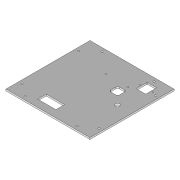
# Autodesk Inventor part: BREEZE-M09
Saved by Autodesk Inventor 2020 (Build 240168000, 168)
## iProperties
Created: 2020-04-12
Part Number: BREEZE-M09
Material: Generic
Description: O2 PANEL
Document SubType Name: Modeling
Designer: John K
Density: 1 g/cm^3
Appearance: Default
Author: John K
Autodesk Inventor part; units mm, degrees
ref_plane "YZ Plane" through (0, 0, 0) normal (1, 0, 0) x (0, 1, 0)
ref_plane "XZ Plane" through (0, 0, 0) normal (0, 1, 0) x (-1, 0, 0)
ref_plane "XY Plane" through (0, 0, 0) normal (0, 0, 1) x (1, 0, 0)
sketch "Face" plane through (0, 0, 0) normal (0, 0, 1) x (1, 0, 0)
  circle A0 centre (-193.5381, 230.5) radius 2.6
  arc A1 (-138.5852, 92.5899) -> (-143.835, 97.8397) centre (-143.835, 92.5899) ccw
  line L0 (-158.1352, 97.8397) -> (-143.835, 97.8397)
  line L1 (-138.5852, 92.5899) -> (-138.5852, 78.2897)
  arc A2 (-158.1352, 97.8397) -> (-163.385, 92.5899) centre (-158.1352, 92.5899) ccw
  arc A3 (-163.385, 78.2897) -> (-158.1352, 73.0399) centre (-158.1352, 78.2897) ccw
  line L2 (-240.4851, 240.5) -> (0, 240.5)
  line L3 (0, 0) -> (0, 240.5)
  line L4 (-240.4851, 240.5) -> (-240.4851, 0)
  line L5 (0, 0) -> (-240.4851, 0)
  circle A4 centre (-10, 42.67) radius 2.6
  arc A5 (-186.2453, 21.7898) -> (-185.2453, 22.7898) centre (-186.2453, 22.7898) ccw
  circle A6 centre (-216.8953, 37.4898) radius 1.7
  line L6 (-212.5453, 22.7898) -> (-212.5453, 52.1898)
  circle A7 centre (-180.8953, 37.4898) radius 1.7
  circle A8 centre (-230.4851, 204.87) radius 2.6
  circle A9 centre (-45, 10) radius 2.6
  line L7 (-185.2453, 52.1898) -> (-185.2453, 22.7898)
  arc A10 (-212.5453, 22.7898) -> (-211.5453, 21.7898) centre (-211.5453, 22.7898) ccw
  line L8 (-68.5351, 195.1795) -> (-120.9351, 195.1795)
  line L9 (-120.9351, 195.1795) -> (-120.9351, 219.9795)
  line L10 (-68.5351, 219.9795) -> (-68.5351, 195.1795)
  line L11 (-120.9351, 219.9795) -> (-68.5351, 219.9795)
  line L12 (-186.2453, 21.7898) -> (-211.5453, 21.7898)
  circle A11 centre (-45, 230.5) radius 2.6
  circle A12 centre (-10, 204.87) radius 2.6
  arc A13 (-185.2453, 52.1898) -> (-186.2453, 53.1898) centre (-186.2453, 52.1898) ccw
  line L13 (-211.5453, 53.1898) -> (-186.2453, 53.1898)
  arc A14 (-211.5453, 53.1898) -> (-212.5453, 52.1898) centre (-211.5453, 52.1898) ccw
  line L14 (-163.385, 78.2897) -> (-163.385, 92.5899)
  line L15 (-143.835, 73.0399) -> (-158.1352, 73.0399)
  circle A15 centre (-230.4851, 42.67) radius 2.6
  circle A16 centre (-193.5381, 10) radius 2.6
  arc A17 (-143.835, 73.0399) -> (-138.5852, 78.2897) centre (-143.835, 78.2897) ccw
  point P0 (-149.3867, 93.8426)
  point P1 (0, 0)
sketch "Sketch1" plane through (0, 0, 0) normal (0, 1, 0) x (-1, 0, 0)
  circle A0 centre (-73.2955, 110.25) radius 2.6
  arc A1 (-18.3426, -27.6601) -> (-23.5924, -22.4103) centre (-23.5924, -27.6601) ccw
  line L0 (-37.8926, -22.4103) -> (-23.5924, -22.4103)
  line L1 (-18.3426, -27.6601) -> (-18.3426, -41.9603)
  arc A2 (-37.8926, -22.4103) -> (-43.1424, -27.6601) centre (-37.8926, -27.6601) ccw
  arc A3 (-43.1424, -41.9603) -> (-37.8926, -47.2101) centre (-37.8926, -41.9603) ccw
  line L2 (-120.2425, 120.25) -> (120.2425, 120.25)
  line L3 (120.2425, -120.25) -> (120.2425, 120.25)
  line L4 (-120.2425, 120.25) -> (-120.2425, -120.25)
  line L5 (120.2425, -120.25) -> (-120.2425, -120.25)
  circle A4 centre (110.2425, -77.58) radius 2.6
  arc A5 (-66.0027, -98.4602) -> (-65.0027, -97.4602) centre (-66.0027, -97.4602) ccw
  circle A6 centre (-96.6527, -82.7602) radius 1.7
  line L6 (-92.3027, -97.4602) -> (-92.3027, -68.0602)
  circle A7 centre (-60.6527, -82.7602) radius 1.7
  circle A8 centre (-110.2425, 84.62) radius 2.6
  circle A9 centre (75.2425, -110.25) radius 2.6
  line L7 (-65.0027, -68.0602) -> (-65.0027, -97.4602)
  arc A10 (-92.3027, -97.4602) -> (-91.3027, -98.4602) centre (-91.3027, -97.4602) ccw
  line L8 (51.7075, 74.9295) -> (-0.6925, 74.9295)
  line L9 (-0.6925, 74.9295) -> (-0.6925, 99.7295)
  line L10 (51.7075, 99.7295) -> (51.7075, 74.9295)
  line L11 (-0.6925, 99.7295) -> (51.7075, 99.7295)
  line L12 (-66.0027, -98.4602) -> (-91.3027, -98.4602)
  circle A11 centre (75.2425, 110.25) radius 2.6
  circle A12 centre (110.2425, 84.62) radius 2.6
  arc A13 (-65.0027, -68.0602) -> (-66.0027, -67.0602) centre (-66.0027, -68.0602) ccw
  line L13 (-91.3027, -67.0602) -> (-66.0027, -67.0602)
  arc A14 (-91.3027, -67.0602) -> (-92.3027, -68.0602) centre (-91.3027, -68.0602) ccw
  line L14 (-43.1424, -41.9603) -> (-43.1424, -27.6601)
  line L15 (-23.5924, -47.2101) -> (-37.8926, -47.2101)
  circle A15 centre (-110.2425, -77.58) radius 2.6
  circle A16 centre (-73.2955, -110.25) radius 2.6
  arc A17 (-23.5924, -47.2101) -> (-18.3426, -41.9603) centre (-23.5924, -41.9603) ccw
  point P0 (0, 0)
  point P1 (-120.2425, 0)
  point P2 (0, 120.25)
  constraints: 1 horizontal alignment, 1 vertical alignment, 2 other
extrude "Extrusion1" add sketch "Sketch1" along normal mid plane 4.75
move faces "Move1" translate (1.5, 0, 0) faces at (-51.7075, -0.7917, 91.4628) (0.6925, 0.7917, 91.4628)
move faces "Move2" translate (13.551, 0, 0) faces at (18.3426, 0.7917, -32.4268) (18.3573, 0.7917, -27.2678) (22.81, 0.7917, -47.1515) (28.3592, -0.7917, -47.2101) (33.1259, -0.7917, -22.4103) (38.6751, 0.7917, -22.4689) (43.1278, 0.7917, -42.3526) (43.1424, -0.7917, -37.1936)
sketch "Sketch2" plane through (0, 2.375, 0) normal (0, 1, 0) x (1, 0, 0)
  line L0 (31.8936, 27.6601) -> (31.8936, 41.9603) projected
  line L1 (2.1925, -74.9295) -> (2.1925, -99.7295) projected
  line L2 (2.1925, -99.7295) -> (2.1925, -74.9295) construction
  line L3 (2.1925, -74.9295) -> (2.1925, 120.25) construction
  line L4 (120.2425, 120.25) -> (-120.2425, 120.25) construction
  line L5 (31.8936, 34.8102) -> (2.1925, 34.8102) construction
  line L6 (48.3962, 60.25) -> (-14.31, 60.25) construction
  point P0 (0, 0)
  point P1 (17.0431, 60.25)
  point P2 (17.0431, 34.8102)
  dimension "d8" = 62.7062
  dimension "d16" = 60
  constraints: 6 end point, 3 midpoint, 2 coincident, 2 point on line, 1 horizontal, 1 perpendicular, 1 vertical, 1 vertical alignment
  measures "d8" distance of L6.start L6.end
  measures "d16" distance between parallel lines of L4 L6
hole "Hole1" at (48.3962, 2.375, -60.25) at (-14.31, 2.375, -60.25) direction (0, -1, 0) diameter 4.5 end through all clearance for "Socket Head Cap Screw" size "M4" standard "Ansi Metric M Profile"
sketch "Sketch3" plane through (0, 2.375, 0) normal (0, 1, 0) x (1, 0, 0)
  line L0 (56.6934, 41.9603) -> (56.6934, 27.6601) projected
  line L1 (91.3027, 67.0602) -> (66.0027, 67.0602) projected
  point P0 (0, 0)
  point P1 (78.6527, 0)
  point P2 (56.6934, 34.8102)
  point P3 (78.6527, 67.0602)
  constraints: 2 midpoint, 1 horizontal alignment, 1 vertical alignment
hole "Hole2" at (78.6527, 2.375, 0) direction (0, -1, 0) diameter 12.7 end through all
body "Solid1"
